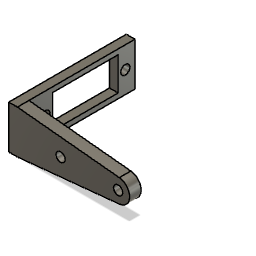
Cam_Servo_Mount v6 (Autodesk Fusion 360 design; units mm, degrees)
Autodesk Fusion 360 part; units mm, degrees
note: some values were not read from the file. Set by a fixed rule: which sketch regions a step uses.
sketch "Skizze1" plane through (0, 0, 0) normal (0, 0, 1) x (1, 0, 0)
  circle A0 centre (-10, 0) radius 1.6
  circle A1 centre (10, 0) radius 1.6
  line L0 (0, 0) -> (0, 16.8871) construction
  arc A2 (10.3958, -3.9804) -> (10.3958, 3.9804) centre (10, 0) ccw
  line L1 (-28, 7.5) -> (-28, -7.5)
  line L2 (10, 0) -> (-66, 0) construction
  line L3 (-25, 7.5) -> (-25, -7.5)
  line L4 (10.3958, 3.9804) -> (-25, 7.5)
  line L5 (10.3958, -3.9804) -> (-25, -7.5)
  line L6 (-25, -7.5) -> (-28, -7.5)
  line L7 (-25, 7.5) -> (-28, 7.5)
  dimension "d1" = 20
  dimension "d2" = 4
  dimension "d3" = 3.2
  dimension "d4" = 28
  dimension "d18" = 15
  dimension "d19" = 3
  constraint coincident L0.start origin
  constraint vertical L0
  constraint symmetric A0 A1 L0
  constraint concentric A1 A2
  constraint horizontal L0.start A0.centre
  constraint vertical L1
  constraint coincident A1.centre A2.centre
  constraint horizontal L2
  constraint midpoint L1 L2
  constraint parallel L1 L3
  constraint tangent A2 L4
  constraint tangent A2 L5
  constraint horizontal L6
  constraint coincident L1 L7.end
  constraint perpendicular L1 L7
  constraint coincident L1.start L7
  measures "d1" distance of A0.centre A1.centre
  measures "d2" radius of A2
  measures "d3" diameter of A1
  measures "d4" distance of L0 L1
  measures "d18" distance of L1.end L1.start
  measures "d19" distance of L1.end L3.end
extrude "Extrusion1" add sketch "Skizze1" along normal blind 4
sketch "Skizze2" plane through (-28, 0, 0) normal (-1, 0, 0) x (0, 0, 1)
  line L0 (0, 7.5) -> (0, -7.5)
  line L1 (4, -7.5) -> (4, 7.5)
  circle A0 centre (-5.75, 0) radius 1.6
  circle A1 centre (-33.5, 0) radius 1.6
  line L2 (-31, -5.75) -> (-31, 5.75)
  line L3 (-31, 5.75) -> (-8.25, 5.75)
  line L4 (-8.25, 5.75) -> (-8.25, -5.75)
  line L5 (-8.25, -5.75) -> (-31, -5.75)
  line L6 (-36.847, 7.5) -> (-36.847, -7.5)
  line L7 (-36.847, -7.5) -> (4, -7.5)
  line L8 (4, -7.5) -> (4, 7.5)
  line L9 (4, 7.5) -> (-36.847, 7.5)
  line L10 (-33.1, 0) -> (0, 0) construction
  circle A2 centre (-25, 0) radius 1.4142 construction
  line L11 (0, -7.5) -> (4, -7.5)
  line L12 (4, 7.5) -> (0, 7.5)
  dimension "d7" = 3.2
  dimension "d8" = 27.75
  dimension "d9" = 19.25
  dimension "d11" = 2.5
  dimension "d12" = 2.5
  dimension "d15" = 25
  dimension "d16" = 15
  dimension "d17" = 11.5
  constraint vertical L2
  constraint perpendicular L2 L3
  constraint perpendicular L3 L4
  constraint perpendicular L2 L5
  constraint perpendicular L5 L6
  constraint perpendicular L6 L7
  constraint perpendicular L7 L8
  constraint horizontal L9
  constraint coincident L10.end origin
  constraint perpendicular L0 L10
  constraint coincident A0.centre L10
  constraint coincident A1.centre L10
  constraint equal A0 A1
  constraint coincident L10 A2.centre
  constraint collinear L1 L8
  constraint symmetric L7 L9 L10
  constraint symmetric L3 L5 L10
  measures "d7" diameter of A1
  measures "d8" distance of A0.centre A1.centre
  measures "d9" distance of A0.centre A2.centre
  measures "d11" distance of A0.centre L4
  measures "d12" distance of A1.centre L2
  measures "d15" distance of L0 A2.centre
  measures "d16" distance of L6.start L6.end
  measures "d17" distance of L3 L5
extrude "Extrusion2" add sketch "Skizze2" against normal blind 3 contours L0 L6 L7 L9
